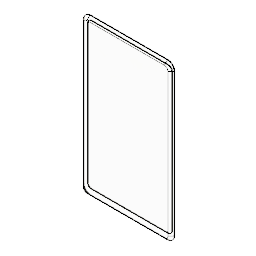
2004745-exact-PANEL, INDICATOR EL (Autodesk Fusion 360 design; units mm, degrees)
Autodesk Fusion 360 part; units mm, degrees
sketch "Sketch1" plane through (0, 0, 0) normal (0, 1, 0) x (1, 0, 0) in component "2004745"
  line L0 (-11.1431, -112.4766) -> (81.2494, -112.4766) construction
  line L1 (-9.4032, -1.7834) -> (86.6433, -1.7834) construction
  line L2 (1.7327, -120.1324) -> (1.7327, 13.1495) construction
  line L3 (66.2487, -119.4365) -> (66.2487, -6.4824) construction
  line L4 (6.4317, -112.4766) -> (61.5497, -112.4766)
  line L5 (66.2487, -107.7776) -> (66.2487, -1.7834)
  line L6 (61.5497, -1.7834) -> (6.4317, -1.7834)
  line L7 (1.7327, -6.4824) -> (1.7327, -107.7776)
  arc A0 (6.4317, -1.7834) -> (1.7327, -6.4824) centre (6.4317, -6.4824) ccw
  arc A1 (66.2487, -6.4824) -> (61.5497, -1.7834) centre (61.5497, -6.4824) ccw
  arc A2 (1.7327, -107.7776) -> (6.4317, -112.4766) centre (6.4317, -107.7776) ccw
  arc A3 (61.5497, -112.4766) -> (66.2487, -107.7776) centre (61.5497, -107.7776) ccw
  line L8 (61.3465, -5.3394) -> (-4.4719, -5.3394) construction
  line L9 (76.7415, -108.9206) -> (-6.2738, -108.9206) construction
  line L10 (4.0949, 11.0388) -> (4.0949, -121.0301) construction
  line L11 (63.8865, 2.5767) -> (63.8865, -121.3323) construction
  line L12 (6.6349, -108.9206) -> (61.3465, -108.9206)
  line L13 (63.8865, -106.3806) -> (63.8865, -7.8794)
  line L14 (63.8865, -5.3394) -> (6.6349, -5.3394)
  line L15 (4.0949, -7.8794) -> (4.0949, -106.3806)
  arc A4 (4.0949, -106.3806) -> (6.6349, -108.9206) centre (6.6349, -106.3806) ccw
  arc A5 (61.3465, -108.9206) -> (63.8865, -106.3806) centre (61.3465, -106.3806) ccw
  arc A6 (6.6349, -5.3394) -> (4.0949, -7.8794) centre (6.6349, -7.8794) ccw
  arc A7 (63.8865, -7.8794) -> (61.3465, -5.3394) centre (61.3465, -7.8794) ccw
  dimension "d1" = 110.6932
  dimension "d2" = 64.516
  dimension "d3" = 4.699
  dimension "d4" = 4.699
  dimension "d5" = 4.699
  dimension "d6" = 4.699
  dimension "d7" = 3.556
  dimension "d8" = 3.556
  dimension "d9" = 2.3622
  dimension "d10" = 2.3622
  dimension "d11" = 2.54
  dimension "d12" = 2.54
  dimension "d13" = 2.54
  dimension "d14" = 2.54
  constraint horizontal L0
  constraint horizontal L1
  constraint perpendicular L0 L2
  constraint perpendicular L1 L3
  constraint horizontal L4
  constraint vertical L5
  constraint horizontal L6
  constraint vertical L7
  constraint coincident L3 L5.end
  constraint coincident L1 L5.end
  constraint tangent L7 A0
  constraint tangent L6 A0
  constraint coincident L5.end L6
  constraint tangent L6 A1
  constraint tangent L3 A1
  constraint tangent L7 A2
  constraint tangent L4 A2
  constraint tangent L4 A3
  constraint tangent L5 A3
  constraint perpendicular L2 L8
  constraint perpendicular L2 L9
  constraint perpendicular L9 L10
  constraint perpendicular L6 L11
  constraint horizontal L12
  constraint vertical L13
  constraint horizontal L14
  constraint vertical L15
  constraint coincident L8 L14.start
  constraint coincident L11 L14.start
  constraint tangent L12 A4
  constraint tangent L15 A4
  constraint tangent L12 A5
  constraint tangent L13 A5
  constraint tangent L15 A6
  constraint tangent L14 A6
  constraint coincident L14.start L13
  constraint tangent L13 A7
  constraint tangent L8 A7
  measures "d1" distance of L0 L1
  measures "d2" distance of L2 L3
  measures "d3" radius of A0
  measures "d4" radius of A1
  measures "d5" radius of A2
  measures "d6" radius of A3
  measures "d7" distance of L1 L8
  measures "d8" distance of L0 L9
  measures "d9" distance of L2 L10
  measures "d10" distance of L3 L11
  measures "d11" radius of A4
  measures "d12" radius of A5
  measures "d13" radius of A6
  measures "d14" radius of A7
extrude "Extrude1" add sketch "Sketch1" along normal blind 0.635 contours L12 L13 L14 L15 A4 A5 A6 A7 in component "2004745"
extrude "Extrude2" add sketch "Sketch1" against normal blind 2.7686 contours L4 L5 L6 L7 A0 A1 A2 A3 | L12 L13 L14 L15 A4 A5 A6 A7 in component "2004745"
chamfer "Chamfer1" distance 2.159 angle 45 8 edges at (33.9907, -2.7686, 1.7834) (64.8723, -2.7686, 3.1597) (66.2487, -2.7686, 57.13) (64.8723, -2.7686, 111.1003) (33.9907, -2.7686, 112.4766) (3.109, -2.7686, 111.1003) (1.7327, -2.7686, 57.13) (3.109, -2.7686, 3.1597) in component "2004745"
component "2004745" placed x (1, 0, 0) y (0, 1, 0) z (0, 0, 1) at (0, 0, 0)
equation "d17 = -0.134 in + 0.025 in"
